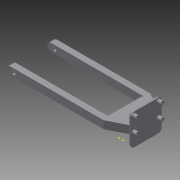
# Autodesk Inventor part: robotCameraArm
Saved by Autodesk Inventor 2015 (Build 190159000, 159)
## iProperties
Created: 2015-02-09
Part Number: robotCameraArm
Material: Generic
Document SubType Name: Modeling
Designer: Gus
Density: 1 g/cm^3
Appearance: Default
Author: Gus
Autodesk Inventor part; units mm, degrees
ref_plane "YZ Plane" through (0, 0, 0) normal (1, 0, 0) x (0, 1, 0)
ref_plane "XZ Plane" through (0, 0, 0) normal (0, 1, 0) x (-1, 0, 0)
ref_plane "XY Plane" through (0, 0, 0) normal (0, 0, 1) x (1, 0, 0)
sketch "Sketch1" plane through (0, 0, 0) normal (0, 1, 0) x (-1, 0, 0)
  line L0 (0, 0) -> (92.075, 0)
  line L1 (92.075, 0) -> (92.075, -4.7714)
  line L2 (92.075, -4.7714) -> (15.875, -4.7714)
  line L3 (15.875, -4.7714) -> (15.875, -33.3464)
  line L4 (15.875, -33.3464) -> (92.075, -33.3464)
  line L5 (92.075, -33.3464) -> (92.075, -38.1089)
  line L6 (92.075, -38.1089) -> (0, -38.1089)
  line L7 (0, -38.1089) -> (0, 0)
  dimension "d0" = 92.075
  dimension "d1" = 4.7714
  dimension "d2" = 76.2
  dimension "d3" = 28.575
  dimension "d4" = 4.7625
  dimension "d5" = 92.075
  constraints: 16 end point, 5 perpendicular, 2 horizontal, 1 vertical
  measures "d0" distance of L0.start L0.end
  measures "d1" distance of L0.end L1.end
  measures "d2" distance of L1.end L2.end
  measures "d3" distance of L2.end L3.end
  measures "d4" distance of L4.end L5.end
  measures "d5" distance from line of L7 L4.end
extrude "Extrusion1" add sketch "Sketch1" along normal blind 6.35
sketch "Sketch2" plane through (-92.075, 0, 0) normal (0, 0, 1) x (1, 0, 0)
  line L0 (7.3295, 3.175) -> (6.4496, 1.651)
  line L1 (6.4496, 1.651) -> (4.6899, 1.651)
  line L2 (4.6899, 1.651) -> (3.81, 3.175)
  line L3 (3.81, 3.175) -> (4.6899, 4.699)
  line L4 (4.6899, 4.699) -> (6.4496, 4.699)
  line L5 (6.4496, 4.699) -> (7.3295, 3.175)
  line L6 (92.075, 0) -> (0, 0) projected
  line L7 (0, 6.35) -> (92.075, 6.35) projected
  line L8 (0, 0) -> (0, 6.35) projected
  point P0 (5.5698, 3.175)
  dimension "d8" = 3.048
  dimension "d10" = 1.651
  dimension "d11" = 3.81
  constraints: 12 end point, 2 parallel, 13 other
  measures "d8" distance between parallel lines of L4 L1
  measures "d10" distance between parallel lines of L7 L4
  measures "d11" distance from line of L8 L2.end
extrude "Extrusion2" cut sketch "Sketch2" against normal blind 43.18
sketch "Sketch3" plane through (0, 0, 0) normal (1, 0, 0) x (0, 0, -1)
  point P0 (0, 0)
sketch "Sketch4" plane through (0, 0, 0) normal (1, 0, 0) x (0, 0, -1)
  line L0 (6.3589, -9.525) -> (6.3589, 15.875)
  line L1 (6.3589, 15.875) -> (31.7589, 15.875)
  line L2 (31.7589, 15.875) -> (31.7589, -9.525)
  line L3 (31.7589, -9.525) -> (6.3589, -9.525)
  line L4 (38.1089, 0) -> (38.1089, 6.35) projected
  line L5 (0, 6.35) -> (38.1089, 6.35) projected
  point P0 (0, 0)
  dimension "d14" = 25.4
  dimension "d15" = 25.4
  dimension "d16" = 25.4
  dimension "d17" = 6.35
  dimension "d18" = 9.525
  constraints: 8 end point, 2 perpendicular, 1 vertical
  measures "d14" distance of L0.start L0.end
  measures "d15" distance of L0.end L1.end
  measures "d16" distance of L1.end L2.end
  measures "d17" distance between parallel lines of L4 L2
  measures "d18" distance between parallel lines of L1 L5
extrude "Extrusion3" add sketch "Sketch4" along normal blind 3.175
sketch "Sketch5" plane through (0, 6.35, 0) normal (0, 1, 0) x (1, 0, 0)
  line L0 (0, 0) -> (-12.7, 0)
  line L1 (-92.075, 0) -> (0, 0) projected
  line L2 (-12.7, 0) -> (0, 6.3589)
  line L3 (0, 6.3589) -> (0, 0)
  line L4 (0, 0) -> (0, 6.3589) projected
  dimension "d21" = 12.7
  constraints: 6 end point, 1 collinear, 1 point on line
  measures "d21" distance of L0.start L0.end
extrude "Extrusion4" cut sketch "Sketch5" against normal blind 6.35
sketch "Sketch6" plane through (0, 6.35, 0) normal (0, 1, 0) x (1, 0, 0)
  line L0 (0, 31.7589) -> (0, 38.1089)
  line L1 (-92.075, 38.1089) -> (0, 38.1089) projected
  line L2 (0, 38.1089) -> (-12.7, 38.1089)
  line L3 (-12.7, 38.1089) -> (0, 31.7589)
  point P0 (0, 0)
  dimension "d24" = 12.7
  constraints: 6 end point, 1 perpendicular, 1 point on line
  measures "d24" distance of L2.end L0.end
extrude "Extrusion5" cut sketch "Sketch6" against normal blind 6.35
sketch "Sketch7" plane through (3.175, 0, 0) normal (1, 0, 0) x (0, 0, -1)
  circle A0 centre (8.8989, 13.335) radius 1.5875
  circle A1 centre (29.2189, 13.335) radius 1.5875
  circle A2 centre (8.8989, 1.5875) radius 1.5875
  circle A3 centre (29.2189, 1.5875) radius 1.5875
  line L0 (6.3589, 15.875) -> (6.3589, -9.525) projected
  line L1 (31.7589, 15.875) -> (6.3589, 15.875) projected
  line L2 (31.7589, -9.525) -> (31.7589, 15.875) projected
  point P0 (0, 0)
  dimension "d27" = 3.175
  dimension "d28" = 3.175
  dimension "d29" = 3.175
  dimension "d30" = 3.175
  dimension "d31" = 2.54
  dimension "d32" = 2.54
  dimension "d33" = 2.54
  dimension "d34" = 2.54
  dimension "d35" = 2.54
  dimension "d36" = 2.54
  dimension "d37" = 14.2875
  dimension "d38" = 14.2875
  constraints: 4 centre point
  measures "d27" diameter of A0
  measures "d28" diameter of A1
  measures "d29" diameter of A2
  measures "d30" diameter of A3
  measures "d31" distance from line of L0 A0.centre
  measures "d32" distance from line of L1 A0.centre
  measures "d33" distance from line of L1 A1.centre
  measures "d34" distance from line of L2 A1.centre
  measures "d35" distance from line of L2 A3.centre
  measures "d36" distance from line of L0 A2.centre
  measures "d37" distance from line of L1 A2.centre
  measures "d38" distance from line of A3.centre L1
extrude "Extrusion6" add sketch "Sketch7" along normal blind 3.175
fillet "Fillet1" radius 3.175 1 edges at (0, 11.1125, -6.3589)
fillet_without_effect "Fillet2"
fillet "Fillet3" radius 3.175 1 edges at (0, 11.1125, -31.7589)
fillet_without_effect "Fillet4"
fillet "Fillet5" radius 3.175 1 edges at (0, -9.525, -19.0589)
fillet "Fillet6" radius 3.175 2 edges at (0, 15.875, -19.0589) (0.9299, 15.875, -30.829)
fillet "Fillet7" radius 3.175 1 edges at (-12.7, 3.175, -38.1089)
fillet "Fillet8" radius 3.175 1 edges at (-12.7, 3.175, 0)
fillet "Fillet9" radius 3.175 1 edges at (-92.075, 6.35, -2.3857)
fillet "Fillet10" radius 3.175 1 edges at (-92.075, 0, -2.3857)
fillet "Fillet11" radius 3.175 1 edges at (-92.075, 6.35, -35.7276)
fillet "Fillet12" radius 3.175 1 edges at (-92.075, 0, -35.7276)
fillet "Fillet13" radius 3.175 1 edges at (-15.875, 6.35, -19.0589)
fillet "Fillet14" radius 3.175 1 edges at (-15.875, 0, -19.0589)
sketch "Sketch8" plane through (6.35, 13.335, -8.8989) normal (1, 0, 0) x (0, 0, -1)
  circle A0 centre (0, 0) radius 1.016
  circle A1 centre (0, 0) radius 1.5875 projected
  circle A2 centre (0, -11.7475) radius 1.016
  circle A3 centre (0, -11.7475) radius 1.5875 projected
  circle A4 centre (20.32, 0) radius 1.016
  circle A5 centre (20.32, 0) radius 1.5875 projected
  circle A6 centre (20.32, -11.7475) radius 1.016
  circle A7 centre (20.32, -11.7475) radius 1.5875 projected
  point P0 (-8.8989, -13.335)
  dimension "d55" = 2.032
  dimension "d56" = 2.032
  dimension "d57" = 2.032
  dimension "d58" = 2.032
  constraints: 4 centre point, 4 concentric
  measures "d55" diameter of A0
  measures "d56" diameter of A2
  measures "d57" diameter of A4
  measures "d58" diameter of A6
extrude "Extrusion7" cut sketch "Sketch8" against normal blind 3.175 contours A0 | A2 | A4 | A6
thread "Thread1" size "2-56 UNC" class "2B" standard "ANSI Unified Screw Threads" full length
thread "Thread2" size "2-56 UNC" class "2B" standard "ANSI Unified Screw Threads" full length
thread "Thread3" size "2-56 UNC" class "2B" standard "ANSI Unified Screw Threads" full length
thread "Thread4" size "2-56 UNC" class "2B" standard "ANSI Unified Screw Threads" full length
sketch "Sketch9" plane through (3.175, 0, 0) normal (1, 0, 0) x (0, 0, -1)
  point P0 (0, 0)
sketch "Sketch10" plane through (3.175, 13.335, -29.2189) normal (1, 0, 0) x (0, 0, -1)
  point P0 (-29.2189, -13.335)
sketch "Sketch11" plane through (3.175, 1.5875, -29.2189) normal (1, 0, 0) x (0, 0, -1)
  point P0 (-29.2189, -1.5875)
body "Solid1"
